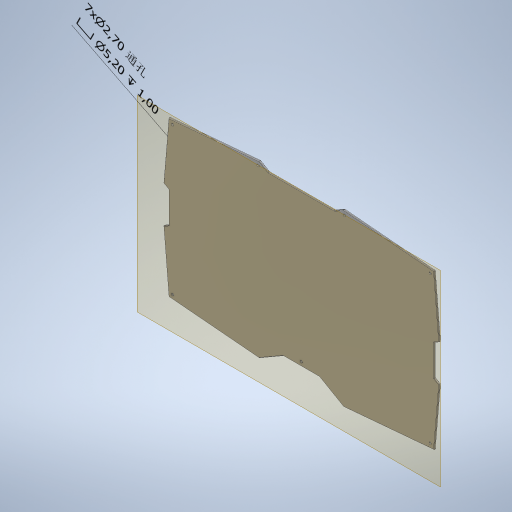
# Autodesk Inventor part: Bottom_Plate
Saved by Autodesk Inventor 2024 (Build 280153000, 153)
## iProperties
Created: 2023-09-20
Part Number: Bottom_Plate
Material: 常规
Document SubType Name: Modeling
Designer: nicx5
Density: 1 g/cm^3
Appearance: 阳极电镀 - 浅灰色
Author: nicx5
Autodesk Inventor part; units mm, degrees
ref_plane "YZ Plane" through (0, 0, 0) normal (1, 0, 0) x (0, 1, 0)
ref_plane "XZ Plane" through (0, 0, 0) normal (0, 1, 0) x (-1, 0, 0)
derived "Frame.ipt"
sketch "bottom面板草图" plane through (-126, -52.8953, -12.6027) normal (0, -0.052336, -0.9986295) x (-1, 0, 0)
  line L0 (-277.9665, 140.9226) -> (-174.3098, 149.979)
  line L1 (-283.8963, 73.2375) -> (-277.9665, 140.9226)
  line L2 (-278, 69.8379) -> (-283.8963, 73.2375)
  line L3 (-278, 34.4886) -> (-278, 69.8379)
  line L4 (-283.8963, 31.089) -> (-278, 34.4886)
  line L5 (-277.9665, -36.5961) -> (-283.8963, 31.089)
  line L6 (-174.3098, -45.6525) -> (-277.9665, -36.5961)
  line L7 (-146.6789, -29.7216) -> (-174.3098, -45.6525)
  line L8 (-105.3211, -29.7216) -> (-146.6789, -29.7216)
  line L9 (-77.6902, -45.6525) -> (-105.3211, -29.7216)
  line L10 (25.9665, -36.5961) -> (-77.6902, -45.6525)
  line L11 (31.8963, 31.089) -> (25.9665, -36.5961)
  line L12 (26.0001, 34.4885) -> (31.8963, 31.089)
  line L13 (26.0001, 69.838) -> (26.0001, 34.4885)
  line L14 (31.8963, 73.2375) -> (26.0001, 69.838)
  line L15 (25.9665, 140.9226) -> (31.8963, 73.2375)
  line L16 (-77.6902, 149.979) -> (25.9665, 140.9226)
  line L17 (-88.0006, 144.0344) -> (-77.6902, 149.979)
  line L18 (-163.9994, 144.0344) -> (-88.0006, 144.0344)
  line L19 (-174.3098, 149.979) -> (-163.9994, 144.0344)
  circle A0 centre (-175.4431, 144.8609) radius 1.5
  circle A1 centre (-273.3518, 136.3068) radius 1.5
  circle A2 centre (-76.5569, 144.8609) radius 1.5
  circle A3 centre (21.3518, 136.3068) radius 1.5
  circle A4 centre (21.3518, -31.9802) radius 1.5
  circle A5 centre (-126, -24.7216) radius 1.5
  circle A6 centre (-273.3518, -31.9802) radius 1.5
  line L20 (-174.3664, 149.7231) -> (-277.7358, 140.6918)
  line L21 (-277.7358, 140.6918) -> (-283.6334, 73.3745)
  line L22 (-283.6334, 73.3745) -> (-277.75, 69.9824)
  line L23 (-277.75, 69.9824) -> (-277.75, 34.3441)
  line L24 (-277.75, 34.3441) -> (-283.6334, 30.952)
  line L25 (-283.6334, 30.952) -> (-277.7358, -36.3653)
  line L26 (-277.7358, -36.3653) -> (-174.3664, -45.3966)
  line L27 (-174.3664, -45.3966) -> (-146.7458, -29.4716)
  line L28 (-146.7458, -29.4716) -> (-105.2542, -29.4716)
  line L29 (-105.2542, -29.4716) -> (-77.6336, -45.3966)
  line L30 (-77.6336, -45.3966) -> (25.7358, -36.3653)
  line L31 (25.7358, -36.3653) -> (31.6334, 30.952)
  line L32 (31.6334, 30.952) -> (25.7501, 34.3441)
  line L33 (25.7501, 34.3441) -> (25.7501, 69.9824)
  line L34 (25.7501, 69.9824) -> (31.6334, 73.3745)
  line L35 (31.6334, 73.3745) -> (25.7358, 140.6918)
  line L36 (25.7358, 140.6918) -> (-77.6336, 149.7231)
  line L37 (-77.6336, 149.7231) -> (-87.9337, 143.7844)
  line L38 (-87.9337, 143.7844) -> (-164.0663, 143.7844)
  line L39 (-164.0663, 143.7844) -> (-174.3664, 149.7231)
  circle A7 centre (-273.3518, 136.3068) radius 2.5
  circle A8 centre (-175.4431, 144.8609) radius 2.5
  circle A9 centre (-76.5569, 144.8609) radius 2.5
  circle A10 centre (21.3518, 136.3068) radius 2.5
  circle A11 centre (21.3518, -31.9897) radius 2.5
  circle A12 centre (-126, -24.7216) radius 2.5
  circle A13 centre (-273.3526, -31.9897) radius 2.5
  point P0 (-126, 52.1633)
extrude "拉伸1" add sketch "bottom面板草图" against normal blind 2 contours A0 | A1 | A2 | A3 | A4 | A5 | A6 | L39 L38 L37 L36 L35 L34 L33 L32 L31 L30 L29 L28 L27 L26 L25 L24 L23 L22 L21 L20 | A7 | A8 | A9 | A10 | A11 | A12 | A13
hole "孔1" at (147.3518, 83.2246, -19.7365) at (49.4431, 91.7671, -20.1842) at (-49.4431, 91.7671, -20.1842) at (-147.3518, 83.2246, -19.7365) at (-147.3518, -84.8317, -10.929) at (0, -77.5831, -11.3089) at (147.3518, -84.8317, -10.929) direction (0, 0.052336, 0.9986295) diameter 2.7 end through all counterbore diameter 5.2 counterbore depth 1
fillet "圆角1" radius 0.5 20 edges at (100.0511, -93.7202, -10.4632) (34.5561, -90.2781, -10.6436) (0, -82.3266, -11.0603) (-34.5561, -90.2781, -10.6436) (-100.0511, -93.7202, -10.4632) (-154.6846, -55.5983, -12.4611) (-154.6918, -20.292, -14.3114) (-151.7501, -0.8036, -15.3328) (-154.6918, 18.6849, -16.3541) (-154.6846, 53.9911, -18.2044) (-100.0511, 92.1131, -20.2023) (-43.2163, 93.6573, -20.2832) (0, 90.6921, -20.1278) (43.2163, 93.6573, -20.2832) (100.0511, 92.1131, -20.2023) (154.6846, 53.9911, -18.2044) (154.6917, 18.6849, -16.3541) (151.75, -0.8036, -15.3328) (154.6917, -20.292, -14.3114) (154.6846, -55.5983, -12.4611)
fillet "圆角2" radius 0.5 20 edges at (-100.0511, 92.2178, -18.2051) (-43.2163, 93.762, -18.286) (0, 90.7967, -18.1306) (43.2163, 93.762, -18.286) (100.0511, 92.2178, -18.2051) (154.6846, 54.0958, -16.2072) (154.6917, 18.7895, -14.3568) (151.75, -0.6989, -13.3355) (154.6917, -20.1873, -12.3142) (154.6846, -55.4936, -10.4638) (100.0511, -93.6156, -8.4659) (34.5561, -90.1734, -8.6463) (0, -82.2219, -9.0631) (-34.5561, -90.1734, -8.6463) (-100.0511, -93.6156, -8.4659) (-154.6846, -55.4936, -10.4638) (-154.6918, -20.1873, -12.3141) (-151.7501, -0.6989, -13.3355) (-154.6918, 18.7896, -14.3568) (-154.6846, 54.0958, -16.2072)
move or copy body "旋转1" bodies to move or copy 1 copy no rotation origin (0, 0, 0) rotation axis (1, 0, 0) rotation angle 3 translate (0, -0.7237, -0.9294)
